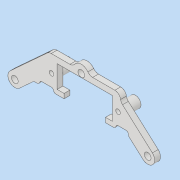
# Autodesk Inventor part: MiniSpoolServoMountBracket
Saved by Autodesk Inventor 2017 (Build 210142000, 142)
## iProperties
Created: 2018-04-09
Part Number: MiniSpoolServoMountBracket
Material: ABS Plastic
Document SubType Name: Modeling
Designer: Derek Wider
Density: 1.06 g/cm^3
Appearance: Smooth - White
Author: Derek Wider
Autodesk Inventor part; units mm, degrees
ref_plane "YZ Plane" through (0, 0, 0) normal (1, 0, 0) x (0, 1, 0)
ref_plane "XZ Plane" through (0, 0, 0) normal (0, 1, 0) x (-1, 0, 0)
ref_plane "XY Plane" through (0, 0, 0) normal (0, 0, 1) x (1, 0, 0)
sketch "Sketch1" plane through (0, 0, 0) normal (0, 0, 1) x (1, 0, 0)
  circle A0 centre (0, 0) radius 1.8415
  circle A1 centre (36.2951, -20.955) radius 1.8415
  circle A2 centre (-36.2951, -20.955) radius 1.8415
  circle A3 centre (-36.2951, -20.955) radius 3.81
  circle A4 centre (36.2951, -20.955) radius 3.81
  line L0 (-36.2951, -20.955) -> (0, 0) construction
  line L1 (0, 0) -> (36.2951, -20.955) construction
  line L2 (0, 0) -> (30.8645, 0) construction
  line L3 (25.7715, -16.637) -> (33.7518, -23.7918)
  line L4 (38.8385, -18.1182) -> (21.463, -2.54)
  line L5 (21.463, -2.54) -> (21.463, 1.27)
  line L6 (17.018, -1.905) -> (-13.208, -1.905)
  line L7 (-17.653, 1.27) -> (-38.8673, -18.1443)
  line L8 (-25.9333, -16.637) -> (-33.7229, -23.7657)
  arc A5 (4.0161, -1.905) -> (-4.0161, -1.905) centre (0, 0) ccw
  line L9 (-4.2597, 1.27) -> (-17.653, 1.27)
  line L10 (4.2597, 1.27) -> (21.463, 1.27)
  line L11 (-13.208, -1.905) -> (-13.208, -14.097)
  line L12 (-13.208, -14.097) -> (-9.398, -14.097)
  line L13 (-9.398, -14.097) -> (-9.398, -16.637)
  line L14 (-9.398, -16.637) -> (-25.9333, -16.637)
  line L15 (17.018, -1.905) -> (17.018, -14.097)
  line L16 (17.018, -14.097) -> (13.208, -14.097)
  line L17 (13.208, -14.097) -> (13.208, -16.637)
  line L18 (13.208, -16.637) -> (25.7715, -16.637)
  dimension "d0" = 3.683
  dimension "d6" = 41.91
  dimension "d7" = 30
  dimension "d8" = 30
  dimension "d9" = 7.62
  dimension "d15" = 4.445
  dimension "d16" = 3.81
  dimension "d24" = 13.208
  dimension "d25" = 12.192
  dimension "d26" = 30.226
  dimension "d27" = 2.54
  dimension "d28" = 3.81
  dimension "d29" = 4.445
  dimension "d30" = 4.445
  dimension "d31" = 3.175
  dimension "d32" = 1.905
  constraints: 38 end point, 8 point on circle, 7 perpendicular, 6 centre point, 5 coincident, 4 horizontal, 4 tangent, 3 equal length, 3 equal radius, 2 horizontal alignment, 2 parallel, 2 point on line, 2 vertical
  measures "d0" diameter of A0
  measures "d6" distance of L0.start L0.end
  measures "d7" angle of L2 L1
  measures "d8" angle of L0 L2
  measures "d9" diameter of A3
  measures "d15" radius of A5
  measures "d16" distance of L5.end L4.end
  measures "d24" distance from line of L11 A5.centre
  measures "d25" distance of L6.end L11.end
  measures "d26" distance of L6.start L6.end
  measures "d27" distance of L12.end L13.end
  measures "d28" distance of L15.end L16.end
  measures "d29" distance between parallel lines of L5 L15
  measures "d30" distance from line of L7.start L11
  measures "d31" distance between parallel lines of L6 L9
  measures "d32" distance from line of L6 point (0, 0)
extrude "Extrusion2" add sketch "Sketch1" along normal blind 3.175
sketch "Sketch2" plane through (0, 0, 3.175) normal (0, 0, 1) x (1, 0, 0)
  line L0 (-25.9333, -16.637) -> (-9.398, -16.637) construction
  line L1 (13.208, -16.637) -> (25.7715, -16.637) construction
  line L2 (-22.733, -16.637) -> (-15.113, -16.637)
  line L3 (-15.113, -16.637) -> (-15.113, -14.605)
  line L4 (-15.113, -14.605) -> (-22.733, -14.605)
  line L5 (-22.733, -14.605) -> (-22.733, -16.637)
  line L6 (18.923, -16.637) -> (25.7715, -16.637)
  line L7 (25.7715, -16.637) -> (25.7715, -14.605)
  line L8 (25.7715, -14.605) -> (18.923, -14.605)
  line L9 (18.923, -14.605) -> (18.923, -16.637)
  line L10 (-13.208, -14.097) -> (-13.208, -1.905) construction
  line L11 (17.018, -1.905) -> (17.018, -14.097) construction
  point P0 (0, 0)
  point P1 (-25.7005, -16.764)
  point P2 (-9.398, -16.637)
  point P3 (23.4202, -16.764)
  dimension "d36" = 1.905
  dimension "d37" = 1.905
  dimension "d38" = 7.62
  dimension "d39" = 2.032
  dimension "d41" = 2.032
  constraints: 16 end point, 4 parallel, 2 horizontal, 2 perpendicular, 4 other
  measures "d36" distance between parallel lines of L10 L3
  measures "d37" distance between parallel lines of L9 L11
  measures "d38" distance of L3.end L4.end
  measures "d39" distance of L2.end L3.end
  measures "d41" distance of L8.end L6.start
extrude "Extrusion3" cut sketch "Sketch2" against normal blind 3.175
fillet "Fillet3" radius 3.175 5 edges at (-4.2597, 1.27, 1.5875) (4.2597, 1.27, 1.5875) (-17.653, 1.27, 1.5875) (21.463, 1.27, 1.5875) (21.463, -2.54, 1.5875)
fillet "Fillet4" radius 1.27 9 edges at (-25.9333, -16.637, 1.5875) (-22.733, -16.637, 1.5875) (-22.733, -14.605, 1.5875) (-15.113, -14.605, 1.5875) (-15.113, -16.637, 1.5875) (18.923, -16.637, 1.5875) (18.923, -14.605, 1.5875) (25.7715, -14.605, 1.5875) (25.7715, -16.637, 1.5875)
sketch "Sketch5" plane through (0, 0, 0) normal (0, 0, -1) x (-1, 0, 0)
  line L0 (-17.018, -1.905) -> (-17.018, -14.097) construction
  line L1 (13.208, -14.097) -> (13.208, -1.905) construction
  circle A0 centre (-20.0787, -8.001) radius 1.27
  circle A1 centre (16.2687, -8.001) radius 1.27
  line L2 (-20.0787, -8.001) -> (-17.018, -8.001) construction
  line L3 (-17.018, -1.905) -> (-17.018, -14.097) construction
  line L4 (16.2687, -8.001) -> (13.208, -8.001) construction
  line L5 (13.208, -14.097) -> (13.208, -1.905) construction
  circle A2 centre (-20.0787, -8.001) radius 3.048
  circle A3 centre (16.2687, -8.001) radius 3.048
  point P0 (0, 0)
  dimension "d52" = 2.54
  dimension "d53" = 36.3474
  dimension "d54" = 6.096
  constraints: 4 centre point, 4 end point, 2 coincident, 2 equal radius, 2 horizontal alignment, 2 midpoint, 1 collinear, 1 perpendicular
  measures "d52" diameter of A0
  measures "d53" distance of L4.start L2.start
  measures "d54" diameter of A2
extrude "Extrusion6" add sketch "Sketch5" along normal blind 6.35
sketch "Sketch6" plane through (20.0787, -8.001, 0) normal (0, 0, -1) x (-1, 0, 0)
  circle A0 centre (0, 0) radius 1.27 projected
  circle A1 centre (36.3474, 0) radius 1.27 projected
  point P0 (20.0787, 8.001)
extrude "Extrusion7" cut sketch "Sketch6" against normal through all
body "Solid2"
